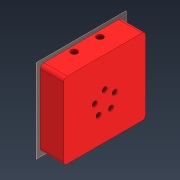
# Autodesk Inventor part: CH_01_0045_endefector_mount
Saved by Autodesk Inventor 2022.3 (Build 263350030, 350C)
## iProperties
Created: 2022-08-15
Part Number: CH_01_0045_endefector_mount
Material: Generic
Document SubType Name: Modeling
Designer: Tomasz Krakowski
Density: 1 g/cm^3
Appearance: Light Red-Orange
Author: Tomasz Krakowski
Autodesk Inventor part; units mm, degrees
ref_plane "XZ Plane" through (0, 0, 0) normal (0, 1, 0) x (-1, 0, 0)
ref_plane "XY Plane" through (0, 0, 0) normal (0, 0, 1) x (1, 0, 0)
sketch "Sketch1" plane through (0, 0, 0) normal (1, 0, 0) x (0, 1, 0)
  line L0 (-25, 25) -> (25, 25) construction
  line L1 (25, 25) -> (25, -25) construction
  line L2 (25, -25) -> (-25, -25) construction
  line L3 (-25, -25) -> (-25, 25) construction
  line L4 (-25, 25) -> (25, -25) construction
  line L5 (25, 25) -> (-25, -25) construction
  circle A0 centre (25, 25) radius 2.25
  circle A1 centre (25, -25) radius 2.25
  circle A2 centre (-25, 25) radius 2.25
  circle A3 centre (-25, -25) radius 2.25
  line L6 (-30, 16) -> (20, 16)
  line L7 (20, 16) -> (20, 0)
  line L8 (20, 0) -> (30, 0) construction
  line L9 (30, 0) -> (30, 30)
  line L10 (30, 30) -> (-30, 30)
  line L11 (-30, 30) -> (-30, 16)
  line L12 (0, 0) -> (20, 0) construction
  line L13 (-30, -16) -> (20, -16)
  line L14 (20, -16) -> (20, 0)
  line L15 (30, 0) -> (30, -30)
  line L16 (30, -30) -> (-30, -30)
  line L17 (-30, -30) -> (-30, -16)
  dimension "d0" = 50
  dimension "d1" = 4.5
  dimension "d2" = 5
  dimension "d3" = 5
  dimension "d4" = 5
  dimension "d5" = 9
  dimension "d6" = 5
  constraints: 36 end point, 6 perpendicular, 4 centre point, 4 coincident, 4 symmetric about line, 3 equal radius, 3 horizontal, 2 midpoint, 2 parallel, 1 collinear
  measures "d0" distance of L0.end L1.end
  measures "d1" diameter of A0
  measures "d2" distance between parallel lines of L10 L0
  measures "d3" distance from line of L11 L0.start
  measures "d4" distance from line of L9 L0.end
  measures "d5" distance from line of L0.start L6
  measures "d6" distance between parallel lines of L1 L7
extrude "Extrusion1" add sketch "Sketch1" along normal blind 20 contours A0 | A1 | A2 | A3 | L11 L10 L9 L15 L16 L17 L13 L14 L7 L6
sketch "Sketch2" plane through (0, 30, 30) normal (0, 1, 0) x (1, 0, 0)
  line L0 (7.5, 0) -> (15.5, 0)
  line L1 (15.5, 0) -> (15.5, 2)
  line L2 (15.5, 2) -> (7.5, 2)
  line L3 (7.5, 2) -> (7.5, 0)
  line L4 (15.5, 0) -> (7.5, 2) construction
  line L5 (0, 0) -> (20, 0) construction
  line L6 (7.5, 58) -> (15.5, 58)
  line L7 (15.5, 58) -> (15.5, 60)
  line L8 (15.5, 60) -> (7.5, 60)
  line L9 (7.5, 60) -> (7.5, 58)
  line L10 (7.5, 58) -> (15.5, 60) construction
  line L11 (15.5, 58) -> (7.5, 60) construction
  line L12 (0, 60) -> (20, 60) construction
  line L13 (0, 0) -> (20, 0) construction
  line L14 (10, 0) -> (11.5, 1) construction
  point P0 (0, 30)
  dimension "d9" = 2
  dimension "d10" = 8
  dimension "d37" = 7.5
  constraints: 24 end point, 5 collinear, 4 parallel, 2 horizontal, 2 midpoint, 2 perpendicular
  measures "d9" distance between parallel lines of L5 L2
  measures "d10" distance between parallel lines of L1 L3
  measures "d37" distance from line of point (0, 30) L3
extrude "Extrusion2" cut sketch "Sketch2" against normal through all
sketch "Sketch3" plane through (20, 0, 0) normal (1, 0, 0) x (0, 0, -1)
  line L0 (-25, -25) -> (25, -25) construction
  line L1 (25, -25) -> (25, 25) construction
  line L2 (25, 25) -> (-25, 25) construction
  line L3 (-25, 25) -> (-25, -25) construction
  line L4 (-25, -25) -> (25, 25) construction
  line L5 (25, -25) -> (-25, 25) construction
  point P0 (0, 0)
  dimension "d13" = 50
  constraints: 12 end point, 4 coincident, 2 midpoint, 2 parallel, 2 perpendicular, 1 horizontal
  measures "d13" distance of L1.end L2.end
hole "Hole1" at (20, 25, 25) at (20, 25, -25) at (20, -25, -25) at (20, -25, 25) direction (-1, 0, 0) diameter 4.2 end through all counterbore diameter 7 counterbore depth 4.1
sketch "Sketch4" plane through (0, 30, 30) normal (0, 1, 0) x (1, 0, 0)
  line L0 (10, 19) -> (10, 41) construction
  line L1 (10, 30) -> (0, 30) construction
  line L2 (0, 60) -> (0, 0) construction
  dimension "d21" = 22
  dimension "d28" = 10
  constraints: 4 end point, 2 perpendicular, 1 midpoint
  measures "d21" distance of L0.start L0.end
  measures "d28" distance of L1.end L1.start
chamfer "Chamfer1" distance 10 angle 45 2 edges at (10, 20, -16) (10, 20, 16)
chamfer "Chamfer2" distance 2 angle 45 2 edges at (15.5, 0, 28) (15.5, 0, -28)
hole "Hole2" at (10, 30, 11) at (10, 30, -11) direction (0, -1, 0) diameter 3.8 end through all
fillet "Fillet1" radius 3 18 edges at (10, 10, 16) (10, 20, 6) (10, 20, -6) (10, 10, -16) (10, -30, -16) (10, -30, 16) (15.5, -30, 29.9999) (17.75, -30, 30) (3.75, -30, 30) (17.75, -30, -30) (15.5, -30, -29.9999) (3.75, -30, -30) (17.75, 30, -30) (15.5, 30, -30) (3.75, 30, -30) (15.5, 30, 30) (17.75, 30, 30) (3.75, 30, 30)
sketch "Sketch5" plane through (0, 30, 27) normal (0, 1, 0) x (1, 0, 0)
  line L0 (25, -8) -> (5, -8)
  line L1 (5, -8) -> (5, 62)
  line L2 (5, 62) -> (25, 62)
  line L3 (25, 62) -> (25, -8)
  line L4 (25, -8) -> (5, 62) construction
  line L5 (5, -8) -> (25, 62) construction
  line L6 (0, 27) -> (15, 27) construction
  line L7 (0, 22.2426) -> (0, 31.7574) construction
  line L8 (20, 54) -> (20, 0) construction
  circle A0 centre (10, 16) radius 1.9 projected
  circle A1 centre (10, 38) radius 1.9 projected
  dimension "d40" = 70
  dimension "d41" = 5
  dimension "d42" = 5
  constraints: 14 end point, 2 midpoint, 2 parallel, 2 perpendicular, 1 horizontal
  measures "d40" distance between parallel lines of L2 L0
  measures "d41" distance from line of L6.start L1
  measures "d42" distance between parallel lines of L8 L3
extrude "Extrusion3" add sketch "Sketch5" along normal blind 5 separate body contours L0 L1 L2 L3 | A0 | A1
sketch "Sketch6" plane through (0, 30, 27) normal (0, -1, 0) x (1, 0, 0)
  line L0 (7.5, 3) -> (7.5, 1) projected
  line L1 (13.5, 1) -> (7.5, 1) projected
  line L2 (7.5, -55) -> (7.5, -57) projected
  line L3 (7.5, -55) -> (13.5, -55) projected
  line L4 (13.5, 3) -> (20, 3)
  line L5 (20, 3) -> (20, -57)
  line L6 (20, -57) -> (13.5, -57)
  line L7 (7.5, 3) -> (5, 3)
  line L8 (5, -62) -> (5, 8) construction
  line L9 (5, 3) -> (5, 8)
  line L10 (7.5, -57) -> (5, -57)
  line L11 (5, -57) -> (5, -62)
  line L12 (5, -62) -> (5, 8) projected
  line L13 (5, 8) -> (25, 8)
  line L14 (25, 8) -> (25, -62) projected
  line L15 (25, 8) -> (25, -62)
  line L16 (25, -62) -> (5, -62) projected
  line L17 (25, -62) -> (5, -62)
  line L18 (13.5, 1) -> (13.5, 3)
  line L19 (13.5, -55) -> (13.5, -57)
  point P0 (0, -27)
  point P1 (20, 0)
  constraints: 24 end point, 5 collinear, 5 perpendicular, 3 horizontal, 1 point on line, 1 vertical
extrude "Extrusion4" add sketch "Sketch6" along normal up to surface (60 mm away) contours L7 L9 L13 L14 L16 L11 L10 L2 L3 L19 L6 L5 L4 L18 L1 L0 bodies 2
fillet "Fillet2" radius 3 4 edges at (15, 35, 35) (15, -30, 35) (15, -30, -35) (15, 35, -35)
chamfer "Chamfer3" distance 2 angle 45 2 edges at (13.5, 0, -30) (13.5, 0, 30)
fillet "Fillet3" radius 3 2 edges at (6.25, 30, -30) (6.25, 30, 30)
sketch "Sketch8" plane through (20, -30, -30) normal (-1, 0, 0) x (0, 0, 1)
  circle A0 centre (30, 30) radius 9 construction
  line L0 (30, 39) -> (30, 30) construction
  point P0 (21.4405, 32.7812)
  point P1 (24.7099, 22.7188)
  point P2 (35.2901, 22.7188)
  point P3 (38.5595, 32.7812)
  dimension "d52" = 18
  dimension "d55" = 360
  constraints: 2 end point, 1 coincident, 1 vertical, 1 vertical alignment, 8 other
hole "Hole3" at (20, 9, 0) at (20, 2.7812, -8.5595) at (20, -7.2812, -5.2901) at (20, -7.2812, 5.2901) at (20, 2.7812, 8.5595) direction (1, 0, 0) diameter 4.2 end through all counterbore diameter 7 counterbore depth 4.1 bodies 2
sketch "Sketch9" plane through (0, 35, 27) normal (0, 1, 0) x (1, 0, 0)
  circle A0 centre (10, 16) radius 1.9 construction
  circle A1 centre (10, 38) radius 1.9 construction
  point P0 (0, 27)
  constraints: 2 coincident
hole "Hole4" at (10, 35, 11) at (10, 35, -11) direction (0, -1, 0) diameter 3.5 end through all counterbore diameter 5.5 counterbore depth 3 bodies 2
ref_plane "Work Plane1" through (5, -29.1213, 34.1213) normal (1, 0, 0) x (0, 1, 0)
sketch "Sketch10" plane through (0, -30, 19) normal (0, -1, 0) x (1, 0, 0)
  line L0 (0, 11) -> (7.5, 11) projected
  line L1 (7.5, 11) -> (7.5, 9) projected
  line L2 (13.5, 9) -> (7.5, 9) projected
  line L3 (13.5, 9) -> (15.5, 11) projected
  line L4 (20, 11) -> (15.5, 11) projected
  line L5 (15.5, -49) -> (20, -49) projected
  line L6 (15.5, -49) -> (13.5, -47) projected
  line L7 (7.5, -47) -> (13.5, -47) projected
  line L8 (7.5, -47) -> (7.5, -49) projected
  line L9 (0, -49) -> (7.5, -49) projected
  line L10 (20, 11) -> (20, -49)
  line L11 (0, -48.8) -> (7.3, -48.8)
  line L12 (7.3, -48.8) -> (7.3, -46.8)
  line L13 (7.3, -46.8) -> (13.5828, -46.8)
  line L14 (13.5828, -46.8) -> (15.5828, -48.8)
  line L15 (15.5828, -48.8) -> (19.8, -48.8)
  line L16 (19.8, -48.8) -> (19.8, 10.8)
  line L17 (19.8, 10.8) -> (15.5828, 10.8)
  line L18 (15.5828, 10.8) -> (13.5828, 8.8)
  line L19 (13.5828, 8.8) -> (7.3, 8.8)
  line L20 (7.3, 8.8) -> (7.3, 10.8)
  line L21 (7.3, 10.8) -> (0, 10.8)
  line L22 (0, 8) -> (0, 11) construction
  line L23 (0, 11) -> (0, 10.8)
  line L24 (0, -49) -> (0, -46) construction
  line L25 (0, -49) -> (0, -48.8)
  line L26 (0, -49) -> (7.5, -49) projected
  point P0 (0, -19)
  dimension "d71" = 0.2
  constraints: 28 end point, 1 collinear, 1 perpendicular, 10 other
  measures "d71" distance between parallel lines of L10 L16
extrude "Extrusion5" cut sketch "Sketch10" against normal through all bodies 1
equation "\"d3\" = d2"
equation "\"d4\" = d2"
equation "\"d6\" = d2"
body "Solid1"
body "Solid2"
